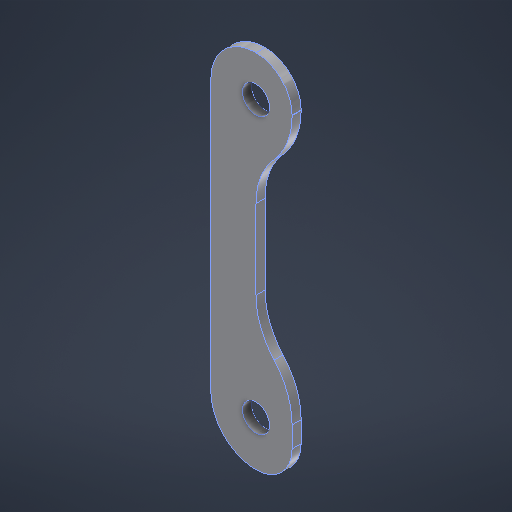
# Autodesk Inventor part: arm1b
Saved by Autodesk Inventor 2025.3 (Build 293356000, 356)
## iProperties
Created: 2016-01-12
Part Number: arm1b
Material: ABS Plastic
Document SubType Name: Modeling
Designer: Nanjar
Density: 1.06 g/cm^3
Appearance: Aluminum - Flat
Author: Nanjar
Autodesk Inventor part; units mm, degrees
ref_plane "YZ Plane" through (0, 0, 0) normal (1, 0, 0) x (0, 1, 0)
ref_plane "XZ Plane" through (0, 0, 0) normal (0, 1, 0) x (-1, 0, 0)
ref_plane "XY Plane" through (0, 0, 0) normal (0, 0, 1) x (1, 0, 0)
sketch "Sketch3" plane through (0, 0, 0) normal (0, 0, 1) x (1, 0, 0)
  circle A0 centre (0, 0) radius 1.5
  circle A1 centre (0, 30.5) radius 1.5
  line L0 (0, 8.5) -> (4, 4.5)
  line L1 (4, 35) -> (4, 25.5)
  line L2 (4, 4.5) -> (4, -5)
  line L3 (0, 21) -> (0, 8.5)
  line L4 (4, 35) -> (-5, 35)
  line L5 (4, -5) -> (-5, -5)
  line L6 (-5, 35) -> (-5, -5)
  line L7 (0, 21) -> (0, 23.5)
  line L8 (4, 25.5) -> (4, 27.5)
  line L9 (4, 27.5) -> (4, 28.5)
  line L10 (4, 27.5) -> (4, 28)
  line L11 (4, 28) -> (0, 23.5)
  dimension "d27" = 40
  dimension "d28" = 4.5
  dimension "d29" = 2.5
  dimension "d32" = 0.5
  constraints: 24 end point, 3 point on line, 2 centre point, 1 coincident, 1 midpoint, 1 vertical
  measures "d27" distance between parallel lines of L5 L4
  measures "d28" distance from line of A1.centre L4
  measures "d29" distance of L3.start L7.end
  measures "d32" distance of L8.end L10.end
extrude "Extrusion2" add sketch "Sketch3" along normal blind 1
fillet "Fillet4" radius 4 2 edges at (4, 35, 0.5) (4, -5, 0.5)
fillet "Fillet6" radius 5 2 edges at (-5, 35, 0.5) (-5, -5, 0.5)
fillet "Fillet7" radius 7.8 4 edges at (0, 23.5, 0.5) (4, 28, 0.5) (0, 8.5, 0.5) (4, 4.5, 0.5)
body "Solid2"
